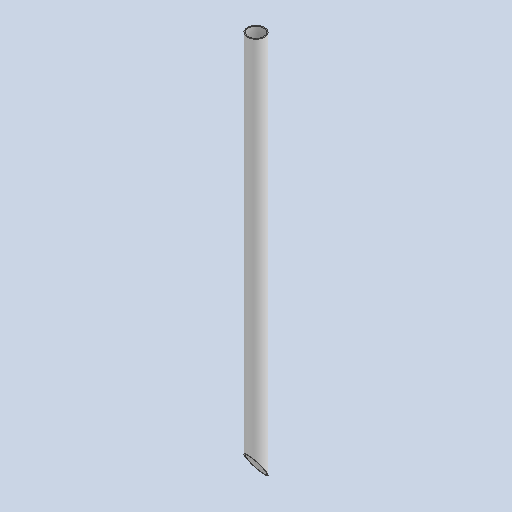
# Autodesk Inventor part: Schräges Rohr CF16
Saved by Autodesk Inventor 2024 (Build 280153000, 153)
## iProperties
Created: 2024-02-28
Part Number: Schräges Rohr CF16
Material: Generisch
Document SubType Name: Modeling
Designer: Andreas Weber
Density: 1 g/cm^3
Appearance: Vorgabe
Mass: 4.64371 g
Surface Area: 94.349 cm^2
Volume: 4.64371 cm^3
Author: Andreas Weber
Autodesk Inventor part; units mm, degrees
ref_plane "YZ Plane" through (0, 0, 0) normal (1, 0, 0) x (0, 1, 0)
ref_plane "XZ Plane" through (0, 0, 0) normal (0, 1, 0) x (-1, 0, 0)
sketch "Skizze1" plane through (0, 0, 0) normal (0, 0, 1) x (1, 0, 0)
  line L0 (-12.6, 0) -> (12.6, 0) construction
  line L1 (0, -12.6) -> (0, 12.6) construction
  circle A0 centre (0, 0) radius 9
  circle A1 centre (0, 0) radius 8
  line L2 (-9, 9) -> (9, 9)
  dimension "d0" = 18
  dimension "d1" = 16
  constraints: 2 centre point, 2 coincident, 2 end point, 1 perpendicular
  measures "d0" diameter of A0
  measures "d1" diameter of A1
extrude "Extrusion4" add sketch "Skizze1" along normal blind 400 contours A0 | A1
extrude "Extrusion5" cut sketch "Skizze1" along normal through all contours A1
ref_plane "Arbeitsebene4" through (-9, 9, 0) normal (0, -0.8333, -0.5529) x (1, 0, 0)
split "Trennen5" plane through (-9, 9, 0) removes the side toward (0, -0.8333, -0.5529)
sketch "Skizze5" plane through (0, 0, 400) normal (0, 0, 1) x (1, 0, 0)
  circle A0 centre (0, 0) radius 8
  circle A1 centre (0, 0) radius 9
  dimension "d17" = 16
  dimension "d18" = 18
  constraints: 2 centre point, 2 coincident
  measures "d17" diameter of A0
  measures "d18" diameter of A1
extrude "Extrusion6" add sketch "Skizze5" along normal blind 5
